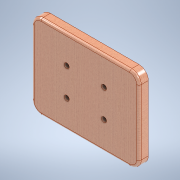
# Autodesk Inventor part: stand
Saved by Autodesk Inventor 2021.1 (Build 251245000, 245)
## iProperties
Created: 2020-08-27
Part Number: stand
Material: Wood (Oak)
Document SubType Name: Sheet Metal
Designer: Vamshi
Mass: 10226.5 g
Surface Area: 6311.38 cm^2
Volume: 13456 cm^3
Density: 0.76 g/cm^3
Sheet Metal Rule: Default
Appearance: White Oak - Natural Medium Gloss
Author: Vamshi
Autodesk Inventor part; units mm, degrees
ref_plane "YZ Plane" through (0, 0, 0) normal (1, 0, 0) x (0, 1, 0)
ref_plane "XZ Plane" through (0, 0, 0) normal (0, 1, 0) x (-1, 0, 0)
ref_plane "XY Plane" through (0, 0, 0) normal (0, 0, 1) x (1, 0, 0)
sketch "Sketch1" plane through (0, 0, 0) normal (0, 0, 1) x (1, 0, 0)
  line L0 (39.2805, 6.8884) -> (521.8805, 6.8884)
  line L1 (572.6805, -43.9116) -> (572.6805, -399.5116)
  line L2 (521.8805, -450.3116) -> (39.2805, -450.3116)
  line L3 (-11.5195, -399.5116) -> (-11.5195, -43.9116)
  arc A0 (-11.5195, -399.5116) -> (39.2805, -450.3116) centre (39.2805, -399.5116) ccw
  arc A1 (39.2805, 6.8884) -> (-11.5195, -43.9116) centre (39.2805, -43.9116) ccw
  arc A2 (572.6805, -43.9116) -> (521.8805, 6.8884) centre (521.8805, -43.9116) ccw
  arc A3 (521.8805, -450.3116) -> (572.6805, -399.5116) centre (521.8805, -399.5116) ccw
  line L4 (280.5805, -450.3116) -> (280.5805, 6.8884)
  line L5 (-11.5195, -221.7116) -> (572.6805, -221.7116)
  circle A4 centre (471.0805, -315.7964) radius 22.86 construction
  circle A5 centre (471.0805, -315.7964) radius 13.97 construction
  circle A6 centre (90.0805, -315.7964) radius 22.86 construction
  circle A7 centre (90.0805, -315.7964) radius 13.97 construction
  circle A8 centre (471.0805, -127.6267) radius 22.86 construction
  circle A9 centre (471.0805, -127.6267) radius 13.97 construction
  circle A10 centre (90.0805, -127.6267) radius 22.86 construction
  circle A11 centre (90.0805, -127.6267) radius 13.97 construction
  point P0 (0, 0)
  point P1 (572.6805, -450.3116)
  point P2 (572.6805, 6.8884)
  point P3 (-11.5195, -450.3116)
  dimension "d0" = 584.2
  dimension "d1" = 457.2
  dimension "d2" = 50.8
  dimension "d3" = 50.8
  dimension "d11" = 45.72
  dimension "d12" = 27.94
  dimension "d13" = 94.0848
  dimension "d14" = 190.5
  constraints: 12 centre point, 12 end point, 8 point on circle, 8 tangent, 6 point on line, 6 symmetric about line, 4 coincident, 4 midpoint, 2 equal radius, 2 parallel, 1 horizontal, 1 perpendicular, 6 other
  measures "d0" distance of point (572.681, -450.312) point (-11.519, -450.312)
  measures "d1" distance of point (572.681, 6.888) point (572.681, -450.312)
  measures "d2" radius of A0
  measures "d3" radius of A1
  measures "d11" diameter of A4
  measures "d12" diameter of A5
  measures "d13" distance from line of L5 A5.centre
  measures "d14" distance from line of L4 A4.centre
extrude "Extrusion1" add sketch "Sketch1" along normal blind 50.8
fillet "Fillet1" radius 12.7 8 edges at (3.3595, -7.9905, 50.8) (-11.5195, -221.7116, 50.8) (3.3595, -435.4326, 50.8) (280.5805, -450.3116, 50.8) (557.8015, -435.4326, 50.8) (572.6805, -221.7116, 50.8) (557.8015, -7.9905, 50.8) (280.5805, 6.8884, 50.8)
sketch "Sketch2" plane through (0, 0, 0) normal (0, 0, -1) x (-1, 0, 0)
  circle A0 centre (-178.9805, -297.9116) radius 22.86
  circle A1 centre (-178.9805, -297.9116) radius 13.97
  line L0 (-521.8805, 6.8884) -> (-39.2805, 6.8884) projected
  line L1 (-280.5805, 6.8884) -> (-280.5805, -454.4869)
  line L2 (-572.6805, -399.5116) -> (-572.6805, -43.9116) projected
  line L3 (-572.6805, -221.7116) -> (11.5195, -221.7116)
  line L4 (11.5195, -43.9116) -> (11.5195, -399.5116) projected
  circle A2 centre (-382.1805, -297.9116) radius 22.86
  circle A3 centre (-382.1805, -297.9116) radius 13.97
  circle A4 centre (-178.9805, -145.5116) radius 22.86
  circle A5 centre (-178.9805, -145.5116) radius 13.97
  circle A6 centre (-382.1805, -145.5116) radius 22.86
  circle A7 centre (-382.1805, -145.5116) radius 13.97
  point P0 (0, 0)
  dimension "d15" = 45.72
  dimension "d16" = 27.94
  dimension "d17" = 76.2
  dimension "d18" = 190.5
  constraints: 8 centre point, 6 symmetric about line, 4 coincident, 4 end point, 3 midpoint, 1 vertical, 6 other
  measures "d15" diameter of A0
  measures "d16" diameter of A1
  measures "d17" distance from line of L3 A0.centre
  measures "d18" distance from line of L4 A0.centre
extrude "Extrusion2" cut sketch "Sketch2" against normal through all contours A1 | A3 | A5 | A7
extrude "Extrusion3" cut sketch "Sketch2" against normal blind 27.94 contours A0 | A2 | A4 | A5 | A6
equation "\"BendRadius\" = Thickness"
equation "\"BendReliefWidth\" = Thickness"
equation "\"BendReliefDepth\" = 0.5 * Thickness"
equation "\"CornerReliefSize\" = 4 * Thickness"
equation "\"MinimumRemnant\" = 2 * Thickness"
equation "\"TransitionRadius\" = BendRadius"
equation "\"JacobiRadiusSize\" = BendRadius"
equation "\"GapSize\" = Thickness"
equation "\"Thickness\" = 3.048"
body "Solid1"
